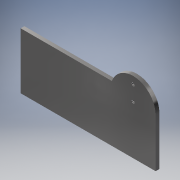
# Autodesk Inventor part: Base
Saved by Autodesk Inventor 2018 (Build 220112000, 112)
## iProperties
Created: 2021-07-05
Part Number: Base
Material: Acero, fundido
Document SubType Name: Modeling
Designer: GABRIEL
Density: 7.85 g/cm^3
Appearance: Semipulido
Author: GABRIEL
Autodesk Inventor part; units mm, degrees
ref_plane "YZ Plane" through (0, 0, 0) normal (1, 0, 0) x (0, 1, 0)
ref_plane "XZ Plane" through (0, 0, 0) normal (0, 1, 0) x (-1, 0, 0)
ref_plane "XY Plane" through (0, 0, 0) normal (0, 0, 1) x (1, 0, 0)
sketch "Boceto2" plane through (0, 0, 0) normal (0, 1, 0) x (-1, 0, 0)
  line L0 (-420, -20) -> (-420, -400)
  line L1 (-420, -400) -> (-60, -400)
  line L2 (-60, -400) -> (-60, 0)
  line L3 (-60, 0) -> (-303.4315, 0)
  arc A0 (-303.4315, 0) -> (-420, -20) centre (-360, -20) ccw
  circle A1 centre (-360, -20) radius 4
  circle A2 centre (-360, 20) radius 4
  dimension "d15" = 360
  dimension "d18" = 60
  dimension "d19" = 8
  dimension "d20" = 8
  dimension "d31" = 60
  dimension "d32" = 40
  dimension "d33" = 60
  dimension "d34" = 400
  constraints: 8 end point, 3 centre point, 3 horizontal, 2 point on circle, 1 coincident, 1 parallel, 1 vertical
  measures "d15" distance of L1.end L0.end
  measures "d18" radius of A0
  measures "d19" diameter of A1
  measures "d20" diameter of A2
  measures "d31" distance from line of L0 A1.centre
  measures "d32" distance of A2.centre A0.centre
  measures "d33" distance from line of L0 A2.centre
  measures "d34" distance of L1.end L2.end
extrude "Extrusión1" add sketch "Boceto2" along normal blind 10
